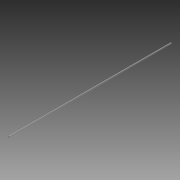
# Autodesk Inventor part: OCT_tubing_25G
Saved by Autodesk Inventor 2011 SP2 (Build 150309200, 309)
## iProperties
Created: 2012-04-17
Part Number: OCT_tubing_25G
Document SubType Name: Modeling
Designer: sungwook
Density: 1 g/cm^3
Author: sungwook
Autodesk Inventor part; units mm, degrees
ref_plane "YZ Plane" through (0, 0, 0) normal (1, 0, 0) x (0, 1, 0)
ref_plane "XZ Plane" through (0, 0, 0) normal (0, 1, 0) x (-1, 0, 0)
ref_plane "XY Plane" through (0, 0, 0) normal (0, 0, 1) x (1, 0, 0)
sketch "Sketch1" plane through (0, 0, 0) normal (0, 0, 1) x (1, 0, 0)
  circle A0 centre (0, 0) radius 0.254
  circle A1 centre (0, 0) radius 0.127
  dimension "d0" = 0.508
  dimension "d1" = 0.254
  constraints: 2 centre point, 2 coincident
  measures "d0" diameter of A0
  measures "d1" diameter of A1
extrude "Extrusion1" add sketch "Sketch1" along normal blind 65
equation "\"d2\" = OCTd0"
equation "\"OCToffset\" = 14.38"
equation "\"lOCTprobeNom\" = 58.38"
equation "\"OCTd0\" = 65"
equation "\"lAdapter\" = 8.38"
equation "\"dTop\" = 6"
equation "\"lOCTprobeTotal\" = 64.38"
body "Solid1"
